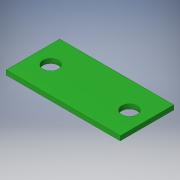
# Autodesk Inventor part: Platine_Gleichrichter
Saved by Autodesk Inventor 2016 (Build 200138000, 138)
## iProperties
Created: 2018-05-16
Part Number: Platine_Gleichrichter
Material: Generic
Document SubType Name: Modeling
Designer: Phil Erle
Density: 1 g/cm^3
Appearance: Smooth - Dark Forest Green
Author: Phil Erle
Autodesk Inventor part; units mm, degrees
ref_plane "YZ Plane" through (0, 0, 0) normal (1, 0, 0) x (0, 1, 0)
ref_plane "XZ Plane" through (0, 0, 0) normal (0, 1, 0) x (-1, 0, 0)
ref_plane "XY Plane" through (0, 0, 0) normal (0, 0, 1) x (1, 0, 0)
sketch "Sketch1" plane through (0, 0, 0) normal (0, 0, 1) x (1, 0, 0)
  line L0 (-20.25, -9.5) -> (20.25, -9.5)
  line L1 (20.25, -9.5) -> (20.25, 9.5)
  line L2 (20.25, 9.5) -> (-20.25, 9.5)
  line L3 (-20.25, 9.5) -> (-20.25, -9.5)
  line L4 (-20.25, -9.5) -> (20.25, 9.5) construction
  line L5 (20.25, -9.5) -> (-20.25, 9.5) construction
  point P0 (0, 0)
  dimension "d0" = 40.5
  dimension "d1" = 19
  constraints: 12 end point, 2 midpoint, 2 parallel, 1 horizontal, 1 perpendicular
  measures "d0" distance of L1.end L2.end
  measures "d1" distance of L0.end L1.end
extrude "Extrusion1" add sketch "Sketch1" along normal blind 1.6
sketch "Sketch2" plane through (0, 0, 1.6) normal (0, 0, 1) x (1, 0, 0)
  line L0 (-14, 0) -> (14, 0) construction
  point P0 (0, 0)
  point P1 (0, 0)
  dimension "d4" = 28
  constraints: 3 coincident, 2 end point, 1 horizontal, 1 horizontal alignment, 1 midpoint
  measures "d4" distance of L0.start L0.end
hole "Hole1" at (-14, 0, 1.6) at (14, 0, 1.6) direction (0, 0, -1) diameter 5.5 depth 8 tip angle 118 clearance for "Countersunk Flat Head Screw DIN EN ISO 2009" size "M5" standard "DIN"
body "Solid1"
